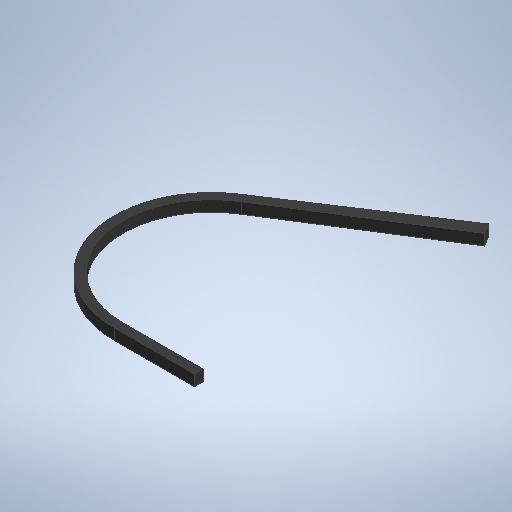
# Autodesk Inventor part: bend_sensor
Saved by Autodesk Inventor 2025.2 (Build 292293000, 293)
## iProperties
Created: 2025-06-25
Part Number: bend_sensor
Material: 一般
Document SubType Name: Modeling
Designer: naka6
Density: 1 g/cm^3
Appearance: 既定
Author: naka6
Autodesk Inventor part; units mm, degrees
ref_plane "YZ Plane" through (0, 0, 0) normal (1, 0, 0) x (0, 1, 0)
ref_plane "XZ Plane" through (0, 0, 0) normal (0, 1, 0) x (-1, 0, 0)
ref_plane "XY Plane" through (0, 0, 0) normal (0, 0, 1) x (1, 0, 0)
sketch "スケッチ1" plane through (0, 0, 0) normal (0, 1, 0) x (-1, 0, 0)
  line L0 (0, 0) -> (-36.8692, 0)
  line L1 (-36.8692, 0) -> (-36.8692, 4.0333)
  line L2 (-36.8692, 4.0333) -> (0, 4.0333)
  line L3 (0, 4.0333) -> (0, 0)
  circle A0 centre (0, -40.6712) radius 40.6712
  circle A1 centre (0, -40.6712) radius 44.7046
  line L4 (22.3684, -74.639) -> (-47.6394, -118.8125)
  line L5 (-47.6394, -118.8125) -> (-44.7046, -123.4637)
  line L6 (-44.7046, -123.4637) -> (24.5213, -78.0504)
  point P0 (21.0303, -75.4832)
  constraints: 14 end point, 2 horizontal, 2 parallel, 2 perpendicular, 2 point on circle, 2 tangent, 1 centre point, 1 coincident, 3 other
extrude "押し出し1" add sketch "スケッチ1" along normal blind 5 contours L0 A1 L3 | L3 A1 L4 A0 | L0 L1 L2 A1 | A1 L6 L5 L4
